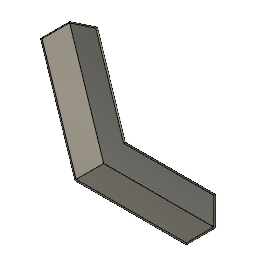
rooftop_support (Autodesk Fusion 360 design; units mm, degrees)
Autodesk Fusion 360 part; units mm, degrees
note: some values were not read from the file. Chosen so that the rebuilt part matches the saved one: which face or edge a step refers to.
box "PrimitivaParallelepipedo1" add length 15 width 60 height 1 placed x (0, 1, 0) y (-1, 0, 0) z (0, 0, 1) at (60, 0, 0) makes body 1
copy_body "CopiaIncollaCorpi1" bodies 1 makes body 2
move_body "Sposta1" bodies 2 to x (1, 0, 0) y (0, 1, 0) z (0, 0, 1) at (0, 0, 1)
move_body "Sposta2" bodies 2 to x (-0.309017, 0, 0.951057) y (0, 1, 0) z (-0.951057, 0, -0.309017) at (0.9511, 0, 1.309)
extrude "Estrusione1" add 1 faces at (-0.317, 10, 0.897) along direction (0.309017, 0, -0.951057) blind 2 on bodies 2 bodies 2 1
split "Dividi1" by plane through (60, 0, 0) normal (0, 0, -1) bodies 2 makes body 3 at (-0.4642, 5, -0.8074)
box "PrimitivaParallelepipedo2" add length 1 width 60 height 15 placed x (0, 1, 0) y (-1, 0, 0) z (0, 0, 1) at (60, 15, 1) separate body makes body 4
copy_body "CopiaIncollaCorpi2" bodies 4 makes body 5
move_body "Sposta3" bodies 5 to x (-0.309017, 0, 0.951057) y (0, 1, 0) z (-0.951057, 0, -0.309017) at (0.9511, 0, 1.309)
move_body "Sposta4" bodies 5 to x (1, 0, 0) y (0, 1, 0) z (0, 0, 1) at (14.2658, 0, 4.6353)
extrude "Estrusione2" add 1 faces at (-6.1803, 15.3333, 20.0211) along direction (-0.951057, 0, -0.309017) blind 1 on bodies 5 bodies 5 2 4
extrude "Estrusione3" add 1 faces at (40, 15.6667, 1) along direction (0, 0, -1) blind 1 on bodies 5 bodies 5
extrude "Estrusione4" add 1 faces at (-0.5592, 15, 0.5637) along direction (0, 1, 0) blind 1 on bodies 5 bodies 5
hidden bodies 3
